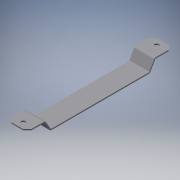
# Autodesk Inventor part: Part106
Saved by Autodesk Inventor 2016 (Build 200138000, 138)
## iProperties
Created: 2018-11-14
Part Number: Part106
Material: Generic
Document SubType Name: Sheet Metal
Designer: hovm
Density: 1 g/cm^3
Sheet Metal Rule: Default_mm
Appearance: Default
Author: hovm
Autodesk Inventor part; units mm, degrees
ref_plane "YZ Plane" through (0, 0, 0) normal (1, 0, 0) x (0, 1, 0)
ref_plane "XZ Plane" through (0, 0, 0) normal (0, 1, 0) x (-1, 0, 0)
ref_plane "XY Plane" through (0, 0, 0) normal (0, 0, 1) x (1, 0, 0)
sketch "Sketch1" plane through (0, 0, 0) normal (0, 0, 1) x (1, 0, 0)
  line L0 (45.8511, 50) -> (65.8511, 50)
  line L1 (65.8511, 50) -> (65.8511, -50)
  line L2 (65.8511, -50) -> (45.8511, -50)
  line L3 (45.8511, -50) -> (45.8511, 50)
  line L4 (45.8511, 50) -> (65.8511, -50) construction
  line L5 (65.8511, 50) -> (45.8511, -50) construction
  line L6 (100.8511, 74.3) -> (100.8511, -74.3)
  point P0 (0, 0)
  point P1 (55.8511, 0)
  point P2 (55.8511, 0)
  dimension "d0" = 100
  dimension "d1" = 20
  dimension "d36" = 45
  measures "d0" distance of L0.end L1.end
  measures "d1" distance of L1.end L2.end
  measures "d36" distance from line of L6 point (55.851, 0)
extrude "Plate1" add sketch "Sketch1" along normal blind 1.2
sketch "Sketch2" plane through (65.8511, -48.9608, 0.6) normal (0, -0.8660254, -0.5) x (1, 0, 0)
  line L0 (-20, 0) -> (0, 0)
  line L1 (0, 0) -> (0, 12)
  line L2 (0, 12) -> (-20, 12)
  line L3 (-20, 12) -> (-20, 0)
  constraints: 6 end point, 1 horizontal, 1 perpendicular, 1 vertical
edge flange "Flange1" height 12 angle 60 thickness 1.2 bend radius 1.2 thickness toward (0, -0.8660254, -0.5) relief tear relief width 1.2 relief depth 0.6 corner gap 1.2 corner form 0 edges at (55.8511, -50, 1.2) (55.8511, 50, 1.2) wall of the first edge with corners at (45.8511, -48.9608, 0.6) (65.8511, -48.9608, 0.6) (65.8511, -54.9608, 10.9923) (45.8511, -54.9608, 10.9923)
bend "Bend1"
corner "Corner1"
sketch "Sketch3" plane through (45.8511, -54.9608, 9.7923) normal (0, 0, 1) x (1, 0, 0)
  line L0 (20, 0) -> (0, 0)
  line L1 (0, 0) -> (0, -18)
  line L2 (0, -18) -> (20, -18)
  line L3 (20, -18) -> (20, 0)
  constraints: 6 end point, 1 horizontal, 1 perpendicular, 1 vertical
edge flange "Flange2" height 18 angle 60 thickness 1.2 bend radius 1.2 thickness toward (0, 0, 1) relief tear relief width 1.2 relief depth 0.6 corner gap 1.2 corner form 0 edges at (55.8511, -56, 10.3923) (55.8511, 56, 10.3923) wall of the first edge with corners at (65.8511, -54.9608, 9.7923) (45.8511, -54.9608, 9.7923) (45.8511, -72.9608, 9.7923) (65.8511, -72.9608, 9.7923)
bend "Bend2"
corner "Corner2"
chamfer "Corner Chamfer1" distance 4 angle 45 4 edges at (45.8511, -72.9608, 10.3923) (65.8511, -72.9608, 10.3923) (45.8511, 72.9608, 10.3923) (65.8511, 72.9608, 10.3923)
sketch "Sketch4" plane through (45.8511, -56.3464, 10.9923) normal (0, 0, 1) x (1, 0, 0)
  line L0 (4, 129.3072) -> (16, 129.3072) projected
  line L1 (16, -16.6144) -> (4, -16.6144) projected
  point P0 (-45.8511, 56.3464)
  point P1 (10, -10.6144)
  point P2 (10, 123.3072)
  point P3 (10, 129.3072)
  point P4 (10, -16.6144)
  dimension "d27" = 6
  dimension "d28" = 6
  constraints: 2 midpoint, 2 vertical alignment
  measures "d27" distance from line of point (10, 123.307) L0
  measures "d28" distance from line of L1 point (10, -10.614)
hole "Hole1" at (55.8511, -66.9608, 10.9923) at (55.8511, 66.9608, 10.9923) direction (0, 0, -1) diameter 4.2 depth 1.2 tip angle 118
equation "\"d34\" = Thickness"
equation "\"d4\" = BendReliefWidth"
equation "\"d5\" = BendReliefDepth"
equation "\"d6\" = MinimumRemnant"
equation "\"d7\" = BendRadius"
equation "\"d10\" = BendRadius"
equation "\"d11\" = CornerReliefSize"
equation "\"d12\" = GapSize"
equation "\"d13\" = JacobiRadiusSize"
equation "\"d14\" = BendReliefWidth"
equation "\"d15\" = BendReliefDepth"
equation "\"d16\" = MinimumRemnant"
equation "\"d17\" = BendRadius"
equation "\"d20\" = BendRadius"
equation "\"d21\" = CornerReliefSize"
equation "\"d22\" = GapSize"
equation "\"d23\" = JacobiRadiusSize"
equation "\"BendRadius\" = Thickness"
equation "\"BendReliefWidth\" = Thickness"
equation "\"BendReliefDepth\" = 0.5 * Thickness"
equation "\"CornerReliefSize\" = 4 * Thickness"
equation "\"MinimumRemnant\" = 2 * Thickness"
equation "\"TransitionRadius\" = BendRadius"
equation "\"JacobiRadiusSize\" = BendRadius"
equation "\"GapSize\" = Thickness"
equation "\"d3\" = BendRadius"
equation "\"Thickness\" = 1.2"
body "Solid1"
